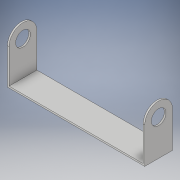
# Autodesk Inventor part: Another Motor Bracket
Saved by Autodesk Inventor 2017 (Build 210142000, 142)
## iProperties
Created: 2017-06-23
Part Number: Another Motor Bracket
Material: Generic
Document SubType Name: Modeling
Designer: Matthew
Density: 1 g/cm^3
Appearance: Default
Author: Matthew
Autodesk Inventor part; units mm, degrees
ref_plane "YZ Plane" through (0, 0, 0) normal (1, 0, 0) x (0, 1, 0)
ref_plane "XZ Plane" through (0, 0, 0) normal (0, 1, 0) x (-1, 0, 0)
ref_plane "XY Plane" through (0, 0, 0) normal (0, 0, 1) x (1, 0, 0)
sketch "Sketch1" plane through (0, 0, 0) normal (1, 0, 0) x (0, 1, 0)
  circle A0 centre (0, 0) radius 14.2875
  line L0 (-66.3768, 26.9875) -> (-66.3768, -26.9875)
  circle A1 centre (0, 0) radius 26.9875
  line L1 (0, 26.9875) -> (-66.3768, 26.9875)
  line L2 (0, -26.9875) -> (-66.3768, -26.9875)
  point P0 (-66.3768, 0)
  dimension "d0" = 28.575
  dimension "d1" = 66.3768
  dimension "d2" = 53.975
  dimension "d3" = 12.7
  constraints: 6 end point, 2 centre point, 2 point on circle, 1 coincident, 1 horizontal, 1 horizontal alignment, 1 midpoint, 1 parallel, 1 vertical
  measures "d0" diameter of A0
  measures "d1" distance from line of point (0, 0) L0
  measures "d2" distance of L0.start L0.end
  measures "d3" radial gap between concentric circles of A0 A1
extrude "Extrusion1" add sketch "Sketch1" along normal blind 3.175
sketch "Sketch2" plane through (0, -66.3768, -26.9875) normal (0, -1, 0) x (1, 0, 0)
  line L0 (0, 0) -> (0, 53.975) projected
  line L1 (0, 53.975) -> (133.35, 53.975)
  line L2 (133.35, 53.975) -> (133.35, 0)
  line L3 (133.35, 0) -> (0, 0)
  line L4 (0, 0) -> (0, 53.975)
  point P0 (0, 26.9875)
  dimension "d6" = 53.975
  dimension "d7" = 133.35
  constraints: 8 end point, 2 parallel, 1 horizontal, 1 perpendicular
  measures "d6" distance of L1.end L2.end
  measures "d7" distance of L2.end L3.end
extrude "Extrusion2" add sketch "Sketch2" along normal blind 3.175
mirror "Mirror1" about plane through (133.35, -66.3768, -26.9875) normal (1, 0, 0)
body "Solid1"
